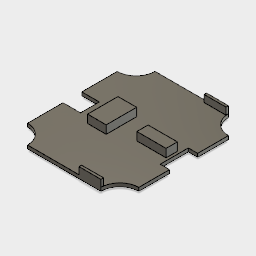
servo_fixer (Autodesk Fusion 360 design; units mm, degrees)
Autodesk Fusion 360 part; units mm, degrees
sketch "スケッチ1" plane through (0, 0, 0) normal (0, 1, 0) x (1, 0, 0)
  line L0 (0, 0) -> (-26.5, 0)
  line L1 (-26.5, 0) -> (-26.5, 54.6)
  line L2 (-26.5, 54.6) -> (0, 54.6)
  line L3 (0, 54.6) -> (0, 0)
  line L4 (0, 54.6) -> (-9.379, 54.6)
  line L5 (-9.379, 54.6) -> (-9.379, 53.506)
  line L6 (-9.379, 53.506) -> (0, 53.506)
  line L7 (0, 53.506) -> (0, 54.6)
  line L8 (0, 0) -> (-9.379, 0)
  line L9 (-9.379, 0) -> (-9.379, 1.094)
  line L10 (-9.379, 1.094) -> (0, 1.094)
  line L11 (0, 1.094) -> (0, 0)
  line L12 (0, 53.506) -> (0, 29.706)
  line L13 (0, 1.094) -> (0, 24.894)
  line L14 (0, 24.894) -> (0, 29.706)
  line L15 (0, 29.706) -> (-9.52, 29.706)
  line L16 (-9.52, 29.706) -> (-9.52, 24.894)
  line L17 (-9.52, 24.894) -> (0, 24.894)
  line L18 (-26.5, 54.6) -> (-26.5, 33.8)
  line L19 (-26.5, 0) -> (-26.5, 20.8)
  line L20 (-26.5, 20.8) -> (-26.5, 33.8)
  line L21 (-26.5, 33.8) -> (-18.529, 33.8)
  line L22 (-18.529, 33.8) -> (-18.529, 20.8)
  line L23 (-18.529, 20.8) -> (-26.5, 20.8)
  line L24 (0, 54.6) -> (8.1, 54.6)
  circle A0 centre (8.1, 54.6) radius 8.1
  line L25 (0, 0) -> (8.1, 0)
  circle A1 centre (8.1, 0) radius 8.1
  line L26 (8.1, 0) -> (8.1, 54.6)
  line L27 (8.1, 0) -> (-39.5, 0)
  line L28 (8.1, 54.6) -> (-39.5, 54.6)
  circle A2 centre (-39.5, 0) radius 8.1
  circle A3 centre (-39.5, 54.6) radius 8.1
  line L29 (-39.5, 0) -> (-39.5, 54.6)
  line L30 (-39.5, 54.6) -> (-39.5, 0)
  line L31 (-39.5, 54.6) -> (-39.5, 27.3)
  line L32 (-39.5, 54.6) -> (-39.5, 27.3)
  line L33 (-39.5, 27.3) -> (-34.5, 27.3)
  line L34 (-32, 23.3) -> (-37, 23.3)
  line L35 (-37, 23.3) -> (-37, 31.3)
  line L36 (-37, 31.3) -> (-32, 31.3)
  line L37 (-32, 31.3) -> (-32, 23.3)
  line L38 (-32, 23.3) -> (-37, 31.3) construction
  line L39 (-37, 23.3) -> (-32, 31.3) construction
  line L40 (8.1, 54.6) -> (8.1, 27.3)
  line L41 (12.1, 21.3) -> (4.1, 21.3)
  line L42 (4.1, 21.3) -> (4.1, 33.3)
  line L43 (4.1, 33.3) -> (12.1, 33.3)
  line L44 (12.1, 33.3) -> (12.1, 21.3)
  line L45 (12.1, 21.3) -> (4.1, 33.3) construction
  line L46 (4.1, 21.3) -> (12.1, 33.3) construction
  dimension "d1" = 26.5
  dimension "d2" = 54.6
  dimension "d5" = 9.379
  dimension "d6" = 1.094
  dimension "d7" = 1.094
  dimension "d8" = 9.379
  dimension "d9" = 23.8
  dimension "d10" = 23.8
  dimension "d11" = 9.52
  dimension "d12" = 20.8
  dimension "d13" = 20.8
  dimension "d14" = 7.971
  dimension "d21" = 8.1
  dimension "d22" = 8.1
  dimension "d27" = 47.6
  dimension "d28" = 47.6
  dimension "d29" = 16.2
  dimension "d30" = 16.2
  dimension "d31" = 5
  dimension "d32" = 5
  dimension "d33" = 8
  dimension "d36" = 12
  dimension "d37" = 8
  constraint horizontal L0
  constraint vertical L1
  constraint horizontal L2
  constraint vertical L3
  constraint horizontal L4
  constraint vertical L5
  constraint horizontal L6
  constraint vertical L7
  constraint horizontal L8
  constraint vertical L9
  constraint horizontal L10
  constraint vertical L11
  constraint perpendicular L14 L15
  constraint parallel L14 L16
  constraint parallel L15 L17
  constraint parallel L12 L14
  constraint perpendicular L20 L21
  constraint parallel L20 L22
  constraint parallel L21 L23
  constraint parallel L18 L20
  constraint coincident A0
  constraint tangent L7 A0
  constraint coincident A1
  constraint tangent L11 A1
  constraint horizontal L28
  constraint perpendicular L28 L29
  constraint perpendicular L27 L30
  constraint midpoint L30
  constraint parallel L31 L32
  constraint perpendicular L34 L35
  constraint parallel L34 L36
  constraint parallel L35 L37
  constraint horizontal L34
  constraint coincident L38
  constraint coincident L39
  constraint midpoint L26
  constraint perpendicular L41 L42
  constraint parallel L41 L43
  constraint parallel L42 L44
  constraint horizontal L41
  constraint coincident L45
  constraint coincident L46
  measures "d29" diameter of A2
  measures "d30" diameter of A3
extrude "押し出し1" add sketch "スケッチ1" against normal blind 1.5 contours L0 L3 L8 L9 L10 L11 L27 | L0 L1 L2 L3 L5 L6 L9 L10 L12 L13 L15 L16 L17 L18 L19 L21 L22 L23 L27 L28 | L3 L14 L15 L16 L17 | L1 L20 L21 L22 L23 | L2 L3 L4 L5 L6 L7 L28
extrude "押し出し2" add sketch "スケッチ1" along normal blind 3.5 contours L3 L14 L15 L16 L17 | L1 L20 L21 L22 L23
extrude "押し出し3" add sketch "スケッチ1" along normal blind 3 contours L0 L3 L8 L9 L10 L11 L27 | L2 L3 L4 L5 L6 L7 L28
extrude "押し出し5" add sketch "スケッチ1" against normal blind 1.5 contours L3 L7 L11 L12 L13 L14 A0 A1 L26 L40 L41 L42 L43
extrude "押し出し6" add 1 faces at (0, 1.1667, -26.498) along direction (1, 0, 0) blind 3
extrude "押し出し7" add sketch "スケッチ1" against normal blind 1.5 contours L1 L18 L19 L20 L27 L28 A2 A3 L29 L30 L31 L32
extrude "押し出し8" cut 1 faces at (-37, -0.5, -25.9667) along direction (-1, 0, 0) blind 2.5
sketch "スケッチ3" plane through (0, -1.5, 0) normal (0, -1, 0) x (1, 0, 0)
  line L0 (-32, -31.3) -> (-39.5, -31.3)
  line L1 (-39.5, -31.3) -> (-39.5, -46.5)
  arc A0 (-31.4, -54.6) -> (-39.5, -46.5) centre (-39.5, -54.6) ccw
  line L2 (-31.4, -54.6) -> (0, -54.6)
  arc A1 (8.1, -46.5) -> (0, -54.6) centre (8.1, -54.6) ccw
  line L3 (8.1, -46.5) -> (8.1, -33.3)
  line L4 (8.1, -33.3) -> (4.1, -33.3)
  line L5 (4.1, -33.3) -> (4.1, -21.3)
  line L6 (4.1, -21.3) -> (8.1, -21.3)
  line L7 (8.1, -21.3) -> (8.1, -8.1)
  arc A2 (0, 0) -> (8.1, -8.1) centre (8.1, 0) ccw
  line L8 (0, 0) -> (-31.4, 0)
  arc A3 (-39.5, -8.1) -> (-31.4, 0) centre (-39.5, 0) ccw
  line L9 (-39.5, -8.1) -> (-39.5, -23.3)
  line L10 (-39.5, -23.3) -> (-32, -23.3)
  line L11 (-32, -23.3) -> (-32, -31.3)
  spline S0 degree 3 poles (-24.2023, -47.412) (-24.2023, -50.948) (-21.325, -53.8255) (-17.7901, -53.8255) knots 0 0 0 0 1 1 1 1
  spline S1 degree 2 poles (-17.7901, -53.8255) (-17.5885, -53.8255) (-8.119, -53.8246) knots 0 0 0 1 1 1
  spline S2 degree 3 poles (-8.119, -53.8246) (-7.7039, -53.8246) (-7.3641, -53.4853) (-7.3641, -53.071) knots 0 0 0 0 1 1 1 1
  line L12 (-7.3641, -53.071) -> (-7.3641, -51.5611)
  spline S3 degree 3 poles (-7.3641, -51.5611) (-7.3641, -51.1468) (-7.7039, -50.8069) (-8.119, -50.8069) knots 0 0 0 0 1 1 1 1
  line L13 (-8.119, -50.8069) -> (-12.3593, -50.8069)
  spline S4 degree 3 poles (-12.3593, -50.8069) (-11.7407, -49.8211) (-11.377, -48.6601) (-11.377, -47.4121) knots 0 0 0 0 1 1 1 1
  spline S5 degree 3 poles (-11.377, -47.4121) (-11.377, -43.8766) (-14.2539, -40.9999) (-17.7901, -40.9999) knots 0 0 0 0 1 1 1 1
  spline S6 degree 3 poles (-17.7901, -40.9999) (-21.325, -40.9998) (-24.2023, -43.8764) (-24.2023, -47.412) knots 0 0 0 0 1 1 1 1
  spline S7 degree 3 poles (-14.3956, -47.412) (-14.3956, -49.2843) (-15.918, -50.8067) (-17.7899, -50.8067) knots 0 0 0 0 1 1 1 1
  spline S8 degree 3 poles (-17.7899, -50.8067) (-19.661, -50.8067) (-21.1835, -49.2844) (-21.1835, -47.412) knots 0 0 0 0 1 1 1 1
  spline S9 degree 3 poles (-21.1835, -47.412) (-21.1835, -45.5414) (-19.661, -44.0187) (-17.7899, -44.0187) knots 0 0 0 0 1 1 1 1
  spline S10 degree 3 poles (-17.7899, -44.0187) (-15.918, -44.0188) (-14.3956, -45.5414) (-14.3956, -47.412) knots 0 0 0 0 1 1 1 1
  line L14 (-8.119, -0.9482) -> (-18.4889, -0.9482)
  spline S11 degree 3 poles (-18.4889, -0.9482) (-21.4015, -0.9482) (-23.7719, -3.3181) (-23.7719, -6.2303) knots 0 0 0 0 1 1 1 1
  line L15 (-23.7719, -6.2303) -> (-23.7719, -8.6396)
  spline S12 degree 3 poles (-23.7719, -8.6396) (-23.7719, -11.5526) (-21.4015, -13.9232) (-18.4889, -13.9232) knots 0 0 0 0 1 1 1 1
  line L16 (-18.4889, -13.9232) -> (-8.119, -13.9232)
  spline S13 degree 3 poles (-8.119, -13.9232) (-7.7039, -13.9232) (-7.3641, -13.5829) (-7.3641, -13.1685) knots 0 0 0 0 1 1 1 1
  line L17 (-7.3641, -13.1685) -> (-7.3641, -11.658)
  spline S14 degree 3 poles (-7.3641, -11.658) (-7.3641, -11.2439) (-7.7039, -10.9053) (-8.119, -10.9053) knots 0 0 0 0 1 1 1 1
  line L18 (-8.119, -10.9053) -> (-18.4889, -10.9053)
  spline S15 degree 3 poles (-18.4889, -10.9053) (-19.7374, -10.9053) (-20.753, -9.8889) (-20.753, -8.6396) knots 0 0 0 0 1 1 1 1
  line L19 (-20.753, -8.6396) -> (-20.753, -6.2304)
  spline S16 degree 3 poles (-20.753, -6.2304) (-20.753, -4.982) (-19.7374, -3.9668) (-18.4889, -3.9668) knots 0 0 0 0 1 1 1 1
  line L20 (-18.4889, -3.9668) -> (-8.119, -3.9664)
  spline S17 degree 3 poles (-8.119, -3.9664) (-7.7039, -3.9664) (-7.3641, -3.627) (-7.3641, -3.2118) knots 0 0 0 0 1 1 1 1
  line L21 (-7.3641, -3.2118) -> (-7.3641, -1.7029)
  spline S18 degree 3 poles (-7.3641, -1.7029) (-7.3641, -1.2877) (-7.7039, -0.9482) (-8.119, -0.9482) knots 0 0 0 0 1 1 1 1
  line L22 (-8.1188, -28.7489) -> (-9.6278, -28.7489)
  spline S19 degree 3 poles (-9.6278, -28.7489) (-10.0425, -28.7489) (-10.382, -29.0887) (-10.382, -29.5036) knots 0 0 0 0 1 1 1 1
  line L23 (-10.382, -29.5036) -> (-10.3825, -33.5053)
  spline S20 degree 3 poles (-10.3825, -33.5053) (-10.3825, -34.7529) (-11.3982, -35.7688) (-12.6465, -35.7688) knots 0 0 0 0 1 1 1 1
  line L24 (-12.6465, -35.7688) -> (-23.0174, -35.7688)
  spline S21 degree 3 poles (-23.0174, -35.7688) (-23.4324, -35.7688) (-23.772, -36.109) (-23.772, -36.5242) knots 0 0 0 0 1 1 1 1
  line L25 (-23.772, -36.5242) -> (-23.772, -38.0325)
  spline S22 degree 3 poles (-23.772, -38.0325) (-23.772, -38.4484) (-23.4324, -38.7874) (-23.0174, -38.7874) knots 0 0 0 0 1 1 1 1
  line L26 (-23.0174, -38.7874) -> (-12.6465, -38.7874)
  spline S23 degree 3 poles (-12.6465, -38.7874) (-9.7336, -38.7874) (-7.3641, -36.4179) (-7.3641, -33.5053) knots 0 0 0 0 1 1 1 1
  line L27 (-7.3641, -33.5053) -> (-7.3641, -29.5036)
  spline S24 degree 3 poles (-7.3641, -29.5036) (-7.3641, -29.0887) (-7.7033, -28.7489) (-8.1188, -28.7489) knots 0 0 0 0 1 1 1 1
  line L28 (-23.772, -17.2875) -> (-23.772, -21.9564)
  spline S25 degree 3 poles (-23.772, -21.9564) (-23.772, -24.8694) (-21.4024, -27.2392) (-18.4898, -27.2392) knots 0 0 0 0 1 1 1 1
  line L29 (-18.4898, -27.2392) -> (-12.6474, -27.2392)
  spline S26 degree 3 poles (-12.6474, -27.2392) (-9.7342, -27.2392) (-7.3641, -24.8694) (-7.3641, -21.9564) knots 0 0 0 0 1 1 1 1
  line L30 (-7.3641, -21.9564) -> (-7.3641, -17.2875)
  spline S27 degree 3 poles (-7.3641, -17.2875) (-7.3641, -16.8721) (-7.7039, -16.5334) (-8.119, -16.5334) knots 0 0 0 0 1 1 1 1
  line L31 (-8.119, -16.5334) -> (-9.6275, -16.5334)
  spline S28 degree 3 poles (-9.6275, -16.5334) (-10.0434, -16.5334) (-10.383, -16.8721) (-10.383, -17.2875) knots 0 0 0 0 1 1 1 1
  line L32 (-10.383, -17.2875) -> (-10.383, -21.9564)
  spline S29 degree 3 poles (-10.383, -21.9564) (-10.383, -23.205) (-11.3985, -24.2205) (-12.6474, -24.2205) knots 0 0 0 0 1 1 1 1
  line L33 (-12.6474, -24.2205) -> (-14.05, -24.2205)
  line L34 (-14.05, -24.2205) -> (-14.05, -17.7063)
  spline S30 degree 3 poles (-14.05, -17.7063) (-14.05, -17.2915) (-14.3902, -16.9522) (-14.8044, -16.9522) knots 0 0 0 0 1 1 1 1
  line L35 (-14.8044, -16.9522) -> (-16.3318, -16.9522)
  spline S31 degree 3 poles (-16.3318, -16.9522) (-16.7462, -16.9522) (-17.086, -17.2915) (-17.086, -17.7063) knots 0 0 0 0 1 1 1 1
  line L36 (-17.086, -17.7063) -> (-17.086, -24.2205)
  line L37 (-17.086, -24.2205) -> (-18.4898, -24.2205)
  spline S32 degree 3 poles (-18.4898, -24.2205) (-19.7377, -24.2205) (-20.7533, -23.205) (-20.7533, -21.9564) knots 0 0 0 0 1 1 1 1
  line L38 (-20.7533, -21.9564) -> (-20.7533, -17.2875)
  spline S33 degree 3 poles (-20.7533, -17.2875) (-20.7533, -16.8721) (-21.0931, -16.5334) (-21.508, -16.5334) knots 0 0 0 0 1 1 1 1
  line L39 (-21.508, -16.5334) -> (-23.0174, -16.5334)
  spline S34 degree 3 poles (-23.0174, -16.5334) (-23.4324, -16.5332) (-23.772, -16.8721) (-23.772, -17.2875) knots 0 0 0 0 1 1 1 1
extrude "押し出し9" add sketch "スケッチ3" along normal blind 1 contours S0 S1 S2 L12 S3 L13 S4 S5 S6 | L14 S11 L15 S12 L16 S13 L17 S14 L18 S15 L19 S16 L20 S17 L21 S18 | L22 S19 L23 S20 L24 S21 L25 S22 L26 S23 L27 S24 | L28 S25 L29 S26 L30 S27 L31 S28 L32 S29 L33 L34 S30 L35 S31 L36 L37 S32 L38 S33 L39 S34
equation "d29 = ( 8.1 * 2 ) * 1 mm"
equation "d30 = ( 8.1 * 2 ) * 1 mm"
